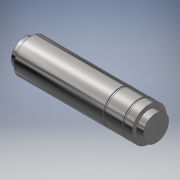
# Autodesk Inventor part: Wheel - Spur Axle
Saved by Autodesk Inventor 2019.4 (Build 234330000, 330)
## iProperties
Created: 2019-11-30
Part Number: Wheel - Spur Axle
Material: Steel, Mild
Document SubType Name: Modeling
Designer: admin
Density: 7.85 g/cm^3
Appearance: Semi-Polished
Author: admin
Autodesk Inventor part; units mm, degrees
ref_plane "YZ Plane" through (0, 0, 0) normal (1, 0, 0) x (0, 1, 0)
ref_plane "XZ Plane" through (0, 0, 0) normal (0, 1, 0) x (-1, 0, 0)
ref_plane "XY Plane" through (0, 0, 0) normal (0, 0, 1) x (1, 0, 0)
sketch "Sketch1" plane through (0, 0, 0) normal (0, 0, 1) x (1, 0, 0)
  line L0 (0, 0) -> (0, 7.5)
  line L1 (0, 7.5) -> (4, 7.5)
  line L2 (4, 7.5) -> (4, 10)
  line L3 (73.2, 10) -> (73.2, 7.5)
  line L4 (73.2, 7.5) -> (77.2, 7.5)
  line L5 (77.2, 7.5) -> (77.2, 0)
  line L6 (77.2, 0) -> (0, 0)
  line L7 (4, 10) -> (56, 10)
  line L8 (56, 10) -> (56, 9.5)
  line L9 (56, 9.5) -> (57.1, 9.5)
  line L10 (57.1, 9.5) -> (57.1, 10)
  line L11 (57.1, 10) -> (67.3, 10)
  line L12 (67.3, 10) -> (67.3, 9.5)
  line L13 (67.3, 9.5) -> (68.4, 9.5)
  line L14 (68.4, 9.5) -> (68.4, 10)
  line L15 (68.4, 10) -> (73.2, 10)
  dimension "d0" = 7.5
  dimension "d2" = 4
  dimension "d3" = 4
  dimension "d4" = 69.2
  dimension "d5" = 52
  dimension "d6" = 0.5
  dimension "d7" = 1.1
  dimension "d8" = 1.1
  dimension "d9" = 10.2
  dimension "d10" = 10
  dimension "d11" = 2.5
  constraints: 32 end point, 9 perpendicular, 7 point on line, 1 collinear, 1 horizontal, 1 vertical
  measures "d0" distance between parallel lines of L6 L1
  measures "d2" distance of L0.end L1.end
  measures "d3" distance of L3.end L4.end
  measures "d4" distance of L2.end L3.start
  measures "d5" distance between parallel lines of L8 L2
  measures "d6" distance of L9.end L10.end
  measures "d7" distance of L8.end L9.end
  measures "d8" distance of L12.end L13.end
  measures "d9" distance between parallel lines of L12 L10
  measures "d10" distance between parallel lines of L6 L7
  measures "d11" distance of L3.start L3.end
revolve "Revolution1" add sketch "Sketch1" angle 360 about axis through (77.2, 0, 0) along (-1, 0, 0)
body "Solid1"
